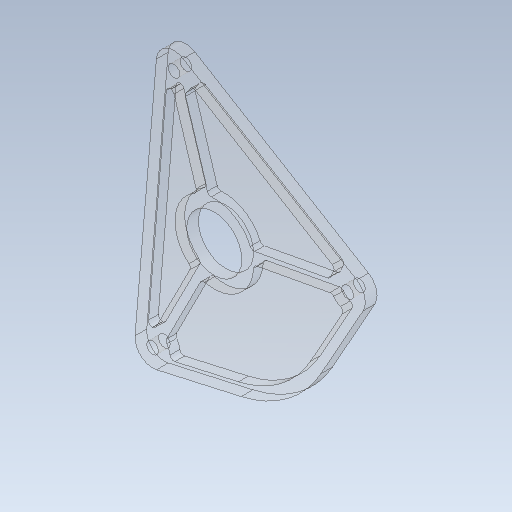
# Autodesk Inventor part: 前足ギアトレイン抑え
Saved by Autodesk Inventor 2020 (Build 240168000, 168)
## iProperties
Created: 2019-10-30
Part Number: 前足ギアトレイン抑え
Material: ポリカーボネート、クリア
Document SubType Name: Modeling
Designer: tanjihayato
Density: 1.2 g/cm^3
Appearance: ポリカーボネート - クリア
Mass: 9.40478 g
Surface Area: 60.5995 cm^2
Volume: 7.83731 cm^3
Author: tanjihayato
Autodesk Inventor part; units mm, degrees
ref_plane "YZ Plane" through (0, 0, 0) normal (1, 0, 0) x (0, 1, 0)
ref_plane "XZ Plane" through (0, 0, 0) normal (0, 1, 0) x (-1, 0, 0)
ref_plane "XY Plane" through (0, 0, 0) normal (0, 0, 1) x (1, 0, 0)
sketch "スケッチ1" plane through (0, 0, 0) normal (0, 0, 1) x (1, 0, 0)
  circle A0 centre (110.4743, -16.4118) radius 30.1 construction
  circle A1 centre (150.4743, 0.5882) radius 1.5
  circle A2 centre (127.6431, 30.2622) radius 1.5
  circle A3 centre (80.4743, 23.124) radius 1.5
  circle A4 centre (70.4743, -10.4118) radius 1.5
  circle A5 centre (110.4743, -16.4118) radius 7.025
  arc A6 (79.801, 27.5733) -> (76.162, 24.4099) centre (80.4743, 23.124) ccw
  arc A7 (131.2097, 33.0062) -> (126.9698, 34.7115) centre (127.6431, 30.2622) ccw
  arc A8 (154.401, -1.6098) -> (154.0408, 3.3323) centre (150.4743, 0.5882) ccw
  arc A9 (66.162, -9.1259) -> (66.7172, -12.8885) centre (70.4743, -10.4118) ccw
  arc A10 (117.3199, -46.749) -> (137.6119, -31.6026) centre (110.4743, -16.4118) ccw
  line L0 (154.401, -1.6098) -> (137.6119, -31.6026)
  line L1 (66.162, -9.1259) -> (76.162, 24.4099)
  line L2 (79.801, 27.5733) -> (126.9698, 34.7115)
  line L3 (131.2097, 33.0062) -> (154.0408, 3.3323)
  line L4 (96.5433, 16.3458) -> (118.2214, -10.0492) construction
  line L5 (117.0311, -23.9953) -> (91.1935, -46.3348) construction
  circle A11 centre (100.1953, 16.6261) radius 3 construction
  circle A12 centre (144.4932, -10.0968) radius 3 construction
  circle A13 centre (100.1953, 16.6261) radius 4.5 construction
  circle A14 centre (144.4932, -10.0968) radius 4.5 construction
  arc A15 (90.988, -49.7066) -> (95.7356, -51.6195) centre (94.7451, -47.2298) ccw
  circle A16 centre (94.7451, -47.2298) radius 3 construction
  line L6 (95.7356, -51.6195) -> (117.3199, -46.749)
  line L7 (66.7172, -12.8885) -> (90.988, -49.7066)
  circle A17 centre (100.1953, 16.6261) radius 1.25
  circle A18 centre (144.4932, -10.0968) radius 1.25
  circle A19 centre (94.7451, -47.2298) radius 1.25
  point P0 (0, 0)
  point P1 (0, 0)
  point P2 (0, 0)
  dimension "d0" = 14.05
  dimension "d1" = 9
  dimension "d2" = 9
  dimension "d3" = 9
  dimension "d4" = 9
  dimension "d5" = 1
  dimension "d6" = 6
  dimension "d7" = 6
  dimension "d8" = 9
  dimension "d9" = 9
  dimension "d10" = 9
  dimension "d11" = 6
  dimension "d12" = 2.5
  dimension "d13" = 2.5
  dimension "d14" = 2.5
  constraints: 20 centre point, 18 tangent, 16 end point, 12 coincident, 12 point on circle
  measures "d0" diameter of A5
  measures "d1" diameter of A6
  measures "d2" diameter of A7
  measures "d3" diameter of A8
  measures "d4" diameter of A9
  measures "d5" radial gap between concentric circles of A10 A0
  measures "d6" diameter of A11
  measures "d7" diameter of A12
  measures "d8" diameter of A13
  measures "d9" diameter of A14
  measures "d10" diameter of A15
  measures "d11" diameter of A16
  measures "d12" diameter of A17
  measures "d13" diameter of A18
  measures "d14" diameter of A19
sketch "スケッチ2" plane through (0, 0, 0) normal (0, 0, 1) x (1, 0, 0)
  circle A0 centre (100.1953, 16.6261) radius 1.25 projected
  circle A1 centre (144.4932, -10.0968) radius 1.25 projected
  circle A2 centre (94.7451, -47.2298) radius 1.25 projected
  line L0 (95.7356, -51.6195) -> (117.3199, -46.749) projected
  arc A3 (117.3199, -46.749) -> (137.6119, -31.6026) centre (110.4743, -16.4118) ccw projected
  line L1 (154.401, -1.6098) -> (137.6119, -31.6026) projected
  arc A4 (90.988, -49.7066) -> (95.7356, -51.6195) centre (94.7451, -47.2298) ccw projected
  arc A5 (102.5197, 20.4792) -> (95.7116, 17.0088) centre (100.1953, 16.6261) ccw
  arc A6 (148.4198, -12.2949) -> (146.8176, -6.2437) centre (144.4932, -10.0968) ccw
  line L2 (148.4198, -12.2949) -> (137.6119, -31.6026)
  arc A7 (90.2614, -46.8472) -> (90.988, -49.7066) centre (94.7451, -47.2298) ccw
  line L3 (90.2614, -46.8472) -> (95.7116, 17.0088)
  line L4 (102.5197, 20.4792) -> (146.8176, -6.2437)
  circle A8 centre (110.4743, -16.4118) radius 7.025 projected
  point P0 (0, 0)
  dimension "d15" = 9
  dimension "d16" = 9
  constraints: 6 end point, 6 point on circle, 5 tangent, 3 centre point, 3 coincident
  measures "d15" diameter of A5
  measures "d16" diameter of A6
extrude "押し出し1" add sketch "スケッチ2" along normal blind 3
sketch "スケッチ3" plane through (0, 0, 3) normal (0, 0, 1) x (1, 0, 0)
  circle A0 centre (110.4743, -16.4118) radius 7.025 projected
  circle A1 centre (94.7451, -47.2298) radius 1.25 projected
  circle A2 centre (144.4932, -10.0968) radius 1.25 projected
  circle A3 centre (100.1953, 16.6261) radius 1.25 projected
  line L0 (95.7356, -51.6195) -> (117.3199, -46.749) projected
  arc A4 (117.3199, -46.749) -> (137.6119, -31.6026) centre (110.4743, -16.4118) ccw projected
  line L1 (137.6119, -31.6026) -> (148.4198, -12.2949) projected
  arc A5 (148.4198, -12.2949) -> (146.8176, -6.2437) centre (144.4932, -10.0968) ccw projected
  line L2 (146.8176, -6.2437) -> (102.5197, 20.4792) projected
  arc A6 (102.5197, 20.4792) -> (95.7116, 17.0088) centre (100.1953, 16.6261) ccw projected
  line L3 (95.7116, 17.0088) -> (90.2614, -46.8472) projected
  arc A7 (90.2614, -46.8472) -> (95.7356, -51.6195) centre (94.7451, -47.2298) ccw projected
  line L4 (100.9701, 17.9105) -> (145.268, -8.8124)
  arc A8 (145.8021, -10.8295) -> (145.268, -8.8124) centre (144.4932, -10.0968) ccw
  line L5 (145.8021, -10.8295) -> (134.9942, -30.1373)
  arc A9 (116.6595, -43.8226) -> (134.9942, -30.1373) centre (110.4743, -16.4118) ccw
  line L6 (116.6595, -43.8226) -> (95.0753, -48.6931)
  arc A10 (93.2506, -47.1023) -> (95.0753, -48.6931) centre (94.7451, -47.2298) ccw
  line L7 (93.2506, -47.1023) -> (98.7007, 16.7536)
  arc A11 (100.9701, 17.9105) -> (98.7007, 16.7536) centre (100.1953, 16.6261) ccw
  circle A12 centre (110.4743, -16.4118) radius 10.025
  arc A13 (98.3399, 12.5264) -> (104.6029, 15.719) centre (100.1953, 16.6261) ccw
  circle A14 centre (144.4932, -10.0968) radius 1.25 projected
  arc A15 (141.6352, -6.6209) -> (143.7297, -14.5316) centre (144.4932, -10.0968) ccw
  arc A16 (99.2139, -47.7592) -> (93.6114, -42.875) centre (94.7451, -47.2298) ccw
  circle A17 centre (94.7451, -47.2298) radius 1.5
  circle A18 centre (144.4932, -10.0968) radius 1.5
  circle A19 centre (100.1953, 16.6261) radius 1.5
  line L8 (110.4743, -16.4118) -> (144.4932, -10.0968) construction
  arc A20 (110.2006, -14.937) -> (110.7481, -17.8866) centre (110.4743, -16.4118) ccw
  arc A21 (144.7669, -11.5716) -> (144.2194, -8.622) centre (144.4932, -10.0968) ccw
  line L9 (100.1953, 16.6261) -> (110.4743, -16.4118) construction
  arc A22 (101.6276, 17.0717) -> (98.763, 16.1804) centre (100.1953, 16.6261) ccw
  arc A23 (109.0421, -16.8574) -> (111.9066, -15.9662) centre (110.4743, -16.4118) ccw
  line L10 (110.4743, -16.4118) -> (94.7451, -47.2298) construction
  arc A24 (111.8104, -17.0937) -> (109.1383, -15.7299) centre (110.4743, -16.4118) ccw
  arc A25 (93.4091, -46.5479) -> (96.0812, -47.9118) centre (94.7451, -47.2298) ccw
  line L11 (110.7481, -17.8866) -> (117.4958, -16.634)
  line L12 (120.4938, -16.0775) -> (140.5956, -12.346)
  line L13 (140.048, -9.3964) -> (119.9462, -13.1279)
  line L14 (116.9483, -13.6844) -> (110.2006, -14.937)
  line L15 (111.9066, -15.9662) -> (109.8677, -9.413)
  line L16 (108.9619, -6.5015) -> (102.888, 13.0206)
  line L17 (100.0234, 12.1294) -> (106.0973, -7.3928)
  line L18 (107.0032, -10.3043) -> (109.0421, -16.8574)
  line L19 (109.1383, -15.7299) -> (108.8606, -16.2741)
  line L20 (104.6322, -24.5586) -> (95.3378, -42.769)
  line L21 (98.0099, -44.1329) -> (107.3043, -25.9224)
  line L22 (108.6904, -23.2065) -> (111.8104, -17.0937)
  point P0 (0, 0)
  point P1 (127.4837, -13.2543)
  point P2 (105.3348, 0.1071)
  point P3 (102.6097, -31.8208)
  dimension "d20" = 3
  dimension "d21" = 3
  dimension "d22" = 3
  dimension "d23" = 3
  dimension "d24" = 3
  dimension "d25" = 3
  dimension "d26" = 3
  dimension "d27" = 3
  dimension "d28" = 3
  dimension "d29" = 3
  dimension "d30" = 3
  constraints: 44 end point, 43 point on circle, 24 tangent, 17 centre point, 12 parallel, 7 point on line, 6 coincident, 3 midpoint, 2 concentric, 7 other
  measures "d20" distance between parallel lines of L2 L4
  measures "d21" radial gap between concentric circles of A0 A12
  measures "d22" diameter of A17
  measures "d23" diameter of A18
  measures "d24" diameter of A19
  measures "d25" radial gap between concentric circles of A13 A19
  measures "d26" radial gap between concentric circles of A15 A18
  measures "d27" radial gap between concentric circles of A16 A17
  measures "d28" diameter of A21
  measures "d29" diameter of A23
  measures "d30" diameter of A25
extrude "押し出し2" cut sketch "スケッチ3" against normal blind 2.5 contours L4 A15 L13 A12 L16 A13 | A13 L17 A12 L20 A16 L7 | A15 L5 A9 L6 A16 L21 A12 L12
extrude "押し出し3" cut sketch "スケッチ3" against normal blind 3 contours A19 A11 | A8 A18 | A17 A10
fillet "フィレット1" radius 1 18 edges at (104.6029, 15.719, 1.75) (102.888, 13.0206, 1.75) (100.0234, 12.1294, 1.75) (98.3399, 12.5264, 1.75) (106.0973, -7.3928, 1.75) (108.9619, -6.5015, 1.75) (119.9462, -13.1279, 1.75) (120.4938, -16.0775, 1.75) (107.3043, -25.9224, 1.75) (104.6322, -24.5586, 1.75) (95.3378, -42.769, 1.75) (93.6114, -42.875, 1.75) (98.0099, -44.1329, 1.75) (99.2139, -47.7592, 1.75) (143.7297, -14.5316, 1.75) (140.5956, -12.346, 1.75) (140.048, -9.3964, 1.75) (141.6352, -6.6209, 1.75)
